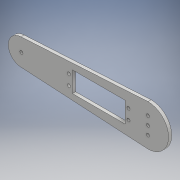
# Autodesk Inventor part: brazo1
Saved by Autodesk Inventor 2018 (Build 220112000, 112)
## iProperties
Created: 2020-03-10
Part Number: brazo1
Material: Genérico
Document SubType Name: Modeling
Designer: sala.ceri
Density: 1 g/cm^3
Appearance: Valor por defecto
Author: sala.ceri
Autodesk Inventor part; units mm, degrees
ref_plane "YZ Plane" through (0, 0, 0) normal (1, 0, 0) x (0, 1, 0)
ref_plane "XZ Plane" through (0, 0, 0) normal (0, 1, 0) x (-1, 0, 0)
ref_plane "XY Plane" through (0, 0, 0) normal (0, 0, 1) x (1, 0, 0)
sketch "Boceto1" plane through (0, 0, 0) normal (0, 1, 0) x (-1, 0, 0)
  arc A0 (120.2602, -12.5039) -> (120.5206, 12.4893) centre (120.13, -0.0046) ccw
  line L0 (21.75, -9.75) -> (71.75, -9.75)
  line L1 (71.75, -9.75) -> (71.75, 9.75)
  line L2 (71.75, 9.75) -> (21.75, 9.75)
  line L3 (21.75, 9.75) -> (21.75, -9.75)
  circle A1 centre (75, 4.875) radius 1.5
  circle A2 centre (75, -4.875) radius 1.5
  circle A3 centre (18.5, 4.875) radius 1.5
  circle A4 centre (18.5, -4.875) radius 1.5
  line L4 (0, 19.5) -> (120.5119, 12.4874)
  line L5 (0, -19.5) -> (119.9998, -12.5039)
  arc A5 (0, 19.5) -> (0, -19.5) centre (0, 0) ccw
  circle A6 centre (120.13, -0.0046) radius 1.5
  circle A7 centre (0, 0) radius 1.5
  circle A8 centre (0, -8) radius 1.5
  circle A9 centre (0, 8) radius 1.5
  line L6 (120.2602, -12.5039) -> (119.9998, -12.5039)
  line L7 (120.5206, 12.4893) -> (120.5119, 12.4874)
  dimension "d107" = 3
  dimension "d108" = 3
  dimension "d110" = 3
  dimension "d112" = 3
  constraints: 16 end point, 10 centre point, 4 point on circle, 2 coincident, 2 perpendicular, 1 horizontal, 1 vertical
  measures "d107" diameter of A6
  measures "d108" diameter of A7
  measures "d110" diameter of A8
  measures "d112" diameter of A9
extrude "Extrusión1" add sketch "Boceto1" along normal blind 3
